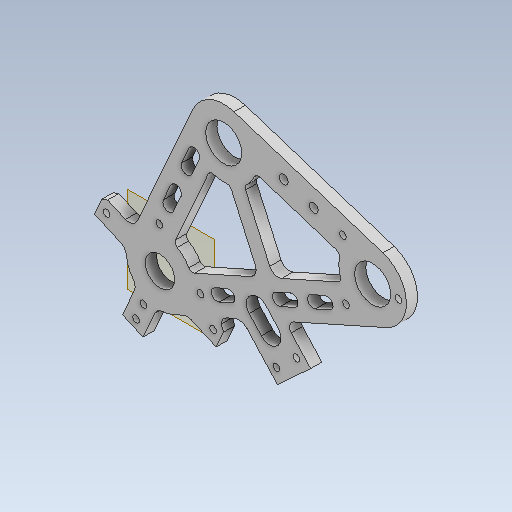
# Autodesk Inventor part: motor_holder_3
Saved by Autodesk Inventor 2020 (Build 240168000, 168)
## iProperties
Created: 2020-05-09
Part Number: motor_holder_3
Material: Generic
Document SubType Name: Modeling
Designer: psrobotics
Density: 1 g/cm^3
Appearance: Default
Author: psrobotics
Autodesk Inventor part; units mm, degrees
ref_plane "YZ Plane" through (0, 0, 0) normal (1, 0, 0) x (0, 1, 0)
ref_plane "XZ Plane" through (0, 0, 0) normal (0, 1, 0) x (-1, 0, 0)
ref_plane "XY Plane" through (0, 0, 0) normal (0, 0, 1) x (1, 0, 0)
ref_plane "Work Plane1" through (0, 0, 3) normal (0, 0, 1) x (1, 0, 0)
sketch "Sketch1" plane through (0, 0, 3) normal (0, 0, 1) x (1, 0, 0)
  circle A0 centre (0, 0) radius 4.075 projected
  circle A1 centre (28.3096, 63.473) radius 5.075 projected
  circle A2 centre (94.4874, 42.242) radius 5.075 projected
  line L0 (0, 0) -> (28.3096, 63.473)
  line L1 (28.3096, 63.473) -> (94.4874, 42.242)
  line L2 (94.4874, 42.242) -> (0, 0)
  line L3 (0, 0) -> (28.3096, 63.473) construction
  line L4 (13.6992, -6.11) -> (42.0088, 57.363)
  line L5 (14.6104, 69.5829) -> (-13.6992, 6.11)
  arc A3 (-13.6992, 6.11) -> (13.6992, -6.11) centre (0, 0) ccw
  arc A4 (42.0088, 57.363) -> (14.6104, 69.5829) centre (28.3096, 63.473) ccw
  line L6 (28.3096, 63.473) -> (94.4874, 42.242) construction
  line L7 (23.7274, 49.19) -> (89.9052, 27.959)
  line L8 (99.0696, 56.525) -> (32.8918, 77.7559)
  arc A5 (32.8918, 77.7559) -> (23.7274, 49.19) centre (28.3096, 63.473) ccw
  arc A6 (89.9052, 27.959) -> (99.0696, 56.525) centre (94.4874, 42.242) ccw
  line L9 (94.4874, 42.242) -> (0, 0) construction
  line L10 (88.3654, 55.9358) -> (-6.122, 13.6938)
  line L11 (6.122, -13.6938) -> (100.6094, 28.5482)
  arc A7 (100.6094, 28.5482) -> (88.3654, 55.9358) centre (94.4874, 42.242) ccw
  arc A8 (-6.122, 13.6938) -> (6.122, -13.6938) centre (0, 0) ccw
  circle A9 centre (0, 0) radius 15
  circle A10 centre (28.3096, 63.473) radius 15
  circle A11 centre (94.4874, 42.242) radius 15
  point P0 (0, 0)
  point P1 (14.1548, 31.7365)
  point P2 (61.3985, 52.8575)
  point P3 (47.2437, 21.121)
  point P4 (13.6938, 6.122)
  point P5 (6.11, 13.6992)
  point P6 (22.1996, 49.7738)
  point P7 (23.7274, 49.19)
  point P8 (42.5926, 58.8907)
  point P9 (80.2044, 46.8242)
  point P10 (80.7936, 36.12)
  point P11 (32.8918, 77.7559)
  point P12 (6.122, -13.6938)
  dimension "d0" = 30
  dimension "d1" = 30
  dimension "d2" = 30
  dimension "d3" = 30
  dimension "d4" = 30
  dimension "d5" = 30
  constraints: 30 end point, 12 point on circle, 12 tangent, 9 centre point, 5 equal length, 3 coincident, 3 midpoint, 1 concentric, 1 point on line
  measures "d0" diameter of A4
  measures "d1" diameter of A6
  measures "d2" diameter of A8
  measures "d3" diameter of A9
  measures "d4" diameter of A10
  measures "d5" diameter of A11
extrude "Extrusion1" add sketch "Sketch1" along normal blind 5 contours A0 L0 L2 | A0 L2 A9 A3 A8 L0 | L2 L0 A0 | A0 L0 A9 L2 | L2 L4 A9 | A9 L10 L0 | L2 L7 A6 L11 A3 L4 | L10 A8 L5 A5 L0 | L2 A11 L7 | A5 A4 L1 A1 L0 | L0 A1 L1 A4 A10 A5 | A11 L1 A2 L2 | L2 A2 L1 A11 A7 A6 | L0 L1 A1 | A1 L1 L0 | L2 L1 A2 | A2 L1 L2 | L1 L10 A11 | L1 A4 L8 A7 L10
sketch "Sketch2" plane through (0, 0, 8) normal (0, 0, 1) x (1, 0, 0)
  line L0 (52.1909, -17.5786) -> (66.9432, -4.074) projected
  line L1 (66.9432, -4.074) -> (60.1909, 3.3021) projected
  line L2 (45.4387, -10.2024) -> (52.1909, -17.5786) projected
  arc A0 (-13.6992, 6.11) -> (6.122, -13.6938) centre (0, 0) ccw projected
  line L3 (6.122, -13.6938) -> (100.6094, 28.5482) projected
  arc A1 (100.6094, 28.5482) -> (99.0696, 56.525) centre (94.4874, 42.242) ccw projected
  line L4 (99.0696, 56.525) -> (32.8918, 77.7559) projected
  arc A2 (32.8918, 77.7559) -> (14.6104, 69.5829) centre (28.3096, 63.473) ccw projected
  line L5 (14.6104, 69.5829) -> (-13.6992, 6.11) projected
  arc A3 (22.1996, 49.7738) -> (42.5926, 58.8907) centre (28.3096, 63.473) ccw projected
  line L6 (42.5926, 58.8907) -> (80.2044, 46.8242) projected
  arc A4 (80.2044, 46.8242) -> (80.7936, 36.12) centre (94.4874, 42.242) ccw projected
  line L7 (80.7936, 36.12) -> (13.6938, 6.122) projected
  arc A5 (13.6938, 6.122) -> (6.11, 13.6992) centre (0, 0) ccw projected
  line L8 (6.11, 13.6992) -> (22.1996, 49.7738) projected
  line L9 (47.4643, -12.4153) -> (36.2889, -0.2073)
  line L10 (6.122, -13.6938) -> (100.6094, 28.5482) projected
  line L11 (62.2166, 1.0892) -> (55.5293, 8.3944)
  circle A6 centre (60.6166, -3.0869) radius 2.05 projected
  circle A7 centre (51.7652, -11.1896) radius 2.05 projected
  line L12 (60.1909, 3.3021) -> (45.4387, -10.2024) projected
  point P0 (0, 0)
  point P1 (36.2889, -0.2073)
  constraints: 4 end point, 2 point on line, 1 parallel
extrude "Extrusion2" add sketch "Sketch2" against normal blind 5 contours L2 L12 L1 L0 | L9 L3 L11 L12 | A6 | A7
sketch "Sketch3" plane through (0, 0, 8) normal (0, 0, 1) x (1, 0, 0)
  circle A0 centre (60.6166, -3.0869) radius 2.05 projected
  circle A1 centre (51.7652, -11.1896) radius 2.05 projected
  point P0 (0, 0)
hole "Hole1" at (60.6166, -3.0869, 8) at (51.7652, -11.1896, 8) direction (0, 0, -1) diameter 3 depth 17
sketch "Sketch4" plane through (0, 0, 8) normal (0, 0, 1) x (1, 0, 0)
  line L0 (-20.0514, 14.2904) -> (-19.0396, 11.6492) projected
  line L1 (-20.0514, 14.2904) -> (-23.2479, 15.7161) projected
  line L2 (-25.8892, 14.7042) -> (-23.2479, 15.7161) projected
  line L3 (-25.8892, 14.7042) -> (-29.1478, 7.3979) projected
  arc A0 (-26.4298, 1.9282) -> (-29.1478, 7.3979) centre (-32.4139, 2.3648) ccw projected
  arc A1 (-26.4298, 1.9282) -> (-18.3105, -19.1566) centre (0, 0) ccw projected
  arc A2 (-16.6845, -25.1334) -> (-18.3105, -19.1566) centre (-22.4562, -23.494) ccw projected
  line L4 (-16.6845, -25.1334) -> (-7.5517, -29.2067) projected
  arc A3 (-2.0186, -26.423) -> (-7.5517, -29.2067) centre (-2.4756, -32.4056) ccw projected
  arc A4 (-2.0186, -26.423) -> (19.0939, -18.3759) centre (0, 0) ccw projected
  arc A5 (24.9796, -16.7435) -> (19.0939, -18.3759) centre (23.4171, -22.5364) ccw projected
  line L5 (24.9796, -16.7435) -> (28.2383, -9.4372) projected
  line L6 (27.2264, -6.796) -> (28.2383, -9.4372) projected
  line L7 (27.2264, -6.796) -> (24.0299, -5.3703) projected
  line L8 (21.3887, -6.3822) -> (24.0299, -5.3703) projected
  line L9 (21.3887, -6.3822) -> (18.5667, -12.7093) projected
  arc A6 (-21.8615, 5.3221) -> (18.5667, -12.7093) centre (0, 0) ccw projected
  line L10 (-21.8615, 5.3221) -> (-19.0396, 11.6492) projected
  circle A7 centre (-23.6864, 10.4368) radius 2.075 projected
  circle A8 centre (23.5915, -10.6496) radius 2.075 projected
  circle A9 centre (-10.5906, -23.7453) radius 2.075 projected
  line L11 (22.2033, -4.5557) -> (29.0529, -7.6107)
  line L12 (29.0529, -7.6107) -> (24.9796, -16.7435)
  line L13 (24.9796, -16.7435) -> (18.13, -13.6885)
  line L14 (18.13, -13.6885) -> (22.2033, -4.5557)
  line L15 (22.2033, -4.5557) -> (24.9796, -16.7435) construction
  line L16 (29.0529, -7.6107) -> (18.13, -13.6885) construction
  circle A10 centre (60.6166, -3.0869) radius 1.5 projected
  circle A11 centre (51.7652, -11.1896) radius 1.5 projected
  line L17 (99.0696, 56.525) -> (32.8918, 77.7559) projected
  arc A12 (32.8918, 77.7559) -> (14.6104, 69.5829) centre (28.3096, 63.473) ccw projected
  line L18 (14.6104, 69.5829) -> (-13.6992, 6.11) projected
  arc A13 (-13.6992, 6.11) -> (6.122, -13.6938) centre (0, 0) ccw projected
  line L19 (6.122, -13.6938) -> (36.2889, -0.2073) projected
  line L20 (36.2889, -0.2073) -> (52.1909, -17.5786) projected
  line L21 (52.1909, -17.5786) -> (66.9432, -4.074) projected
  line L22 (66.9432, -4.074) -> (55.5293, 8.3944) projected
  line L23 (55.5293, 8.3944) -> (100.6094, 28.5482) projected
  arc A14 (100.6094, 28.5482) -> (99.0696, 56.525) centre (94.4874, 42.242) ccw projected
  line L24 (6.11, 13.6992) -> (22.1996, 49.7738) projected
  arc A15 (22.1996, 49.7738) -> (42.5926, 58.8907) centre (28.3096, 63.473) ccw projected
  line L25 (42.5926, 58.8907) -> (80.2044, 46.8242) projected
  arc A16 (80.2044, 46.8242) -> (80.7936, 36.12) centre (94.4874, 42.242) ccw projected
  line L26 (80.7936, 36.12) -> (13.6938, 6.122) projected
  arc A17 (13.6938, 6.122) -> (6.11, 13.6992) centre (0, 0) ccw projected
  line L27 (18.13, -13.6885) -> (12.1249, -11.0101)
  line L28 (6.122, -13.6938) -> (36.2889, -0.2073) projected
  point P0 (0, 0)
  point P1 (28.2382, -9.4374)
  point P2 (24.3854, -5.5289)
  dimension "d17" = 7.5
  dimension "d18" = 10
  constraints: 14 end point, 2 collinear, 2 midpoint, 2 parallel, 1 perpendicular, 1 point on line
  measures "d17" distance of L11.start L11.end
  measures "d18" distance of L11.end L12.end
extrude "Extrusion3" add sketch "Sketch4" against normal blind 5 contours L27 L19 L9 A6 | A6 L14 L27 | L9 L19 L7 L6 L5 L13 L14 | L6 L11 L12
sketch "Sketch5" plane through (0, 0, 8) normal (0, 0, 1) x (1, 0, 0)
  circle A0 centre (-10.5906, -23.7453) radius 2.075 projected
  circle A1 centre (-23.6864, 10.4368) radius 2.075 projected
  line L0 (-20.0514, 14.2904) -> (-19.0396, 11.6492) projected
  line L1 (-20.0514, 14.2904) -> (-23.2479, 15.7161) projected
  line L2 (-25.8892, 14.7042) -> (-23.2479, 15.7161) projected
  line L3 (-25.8892, 14.7042) -> (-29.1478, 7.3979) projected
  arc A2 (-26.4298, 1.9282) -> (-29.1478, 7.3979) centre (-32.4139, 2.3648) ccw projected
  arc A3 (-26.4298, 1.9282) -> (-18.3105, -19.1566) centre (0, 0) ccw projected
  arc A4 (-16.6845, -25.1334) -> (-18.3105, -19.1566) centre (-22.4562, -23.494) ccw projected
  line L4 (-16.6845, -25.1334) -> (-7.5517, -29.2067) projected
  arc A5 (-2.0186, -26.423) -> (-7.5517, -29.2067) centre (-2.4756, -32.4056) ccw projected
  arc A6 (-2.0186, -26.423) -> (19.0939, -18.3759) centre (0, 0) ccw projected
  arc A7 (24.9796, -16.7435) -> (19.0939, -18.3759) centre (23.4171, -22.5364) ccw projected
  line L5 (24.9796, -16.7435) -> (28.2383, -9.4372) projected
  line L6 (27.2264, -6.796) -> (28.2383, -9.4372) projected
  line L7 (27.2264, -6.796) -> (24.0299, -5.3703) projected
  line L8 (21.3887, -6.3822) -> (24.0299, -5.3703) projected
  line L9 (21.3887, -6.3822) -> (18.5667, -12.7093) projected
  arc A8 (-21.8615, 5.3221) -> (18.5667, -12.7093) centre (0, 0) ccw projected
  line L10 (-21.8615, 5.3221) -> (-19.0396, 11.6492) projected
  circle A9 centre (-23.6864, 10.4368) radius 2.075 projected
  circle A10 centre (23.5915, -10.6496) radius 2.075 projected
  circle A11 centre (-10.5906, -23.7453) radius 2.075 projected
  line L11 (-4.4968, -22.3571) -> (-7.5517, -29.2067)
  line L12 (-7.5517, -29.2067) -> (-16.6845, -25.1334)
  line L13 (-16.6845, -25.1334) -> (-13.6296, -18.2838)
  line L14 (-13.6296, -18.2838) -> (-4.4968, -22.3571)
  line L15 (-4.4968, -22.3571) -> (-16.6845, -25.1334) construction
  line L16 (-7.5517, -29.2067) -> (-13.6296, -18.2838) construction
  line L17 (-18.2249, 13.4757) -> (-25.0745, 16.5307)
  line L18 (-25.0745, 16.5307) -> (-29.1478, 7.3979)
  line L19 (-29.1478, 7.3979) -> (-22.2982, 4.3429)
  line L20 (-22.2982, 4.3429) -> (-18.2249, 13.4757)
  line L21 (-18.2249, 13.4757) -> (-29.1478, 7.3979) construction
  line L22 (-25.0745, 16.5307) -> (-22.2982, 4.3429) construction
  circle A12 centre (23.5915, -10.6496) radius 2.075 projected
  circle A13 centre (60.6166, -3.0869) radius 1.5 projected
  circle A14 centre (51.7652, -11.1896) radius 1.5 projected
  line L23 (99.0696, 56.525) -> (32.8918, 77.7559) projected
  arc A15 (32.8918, 77.7559) -> (14.6104, 69.5829) centre (28.3096, 63.473) ccw projected
  line L24 (14.6104, 69.5829) -> (-13.6992, 6.11) projected
  arc A16 (-13.6992, 6.11) -> (6.122, -13.6938) centre (0, 0) ccw projected
  line L25 (6.122, -13.6938) -> (12.1249, -11.0101) projected
  line L26 (12.1249, -11.0101) -> (24.9796, -16.7435) projected
  line L27 (24.9796, -16.7435) -> (29.0529, -7.6107) projected
  line L28 (29.0529, -7.6107) -> (24.3854, -5.5289) projected
  line L29 (24.3854, -5.5289) -> (36.2889, -0.2073) projected
  line L30 (36.2889, -0.2073) -> (52.1909, -17.5786) projected
  line L31 (52.1909, -17.5786) -> (66.9432, -4.074) projected
  line L32 (66.9432, -4.074) -> (55.5293, 8.3944) projected
  line L33 (55.5293, 8.3944) -> (100.6094, 28.5482) projected
  arc A17 (100.6094, 28.5482) -> (99.0696, 56.525) centre (94.4874, 42.242) ccw projected
  line L34 (6.11, 13.6992) -> (22.1996, 49.7738) projected
  arc A18 (22.1996, 49.7738) -> (42.5926, 58.8907) centre (28.3096, 63.473) ccw projected
  line L35 (42.5926, 58.8907) -> (80.2044, 46.8242) projected
  arc A19 (80.2044, 46.8242) -> (80.7936, 36.12) centre (94.4874, 42.242) ccw projected
  line L36 (80.7936, 36.12) -> (13.6938, 6.122) projected
  arc A20 (13.6938, 6.122) -> (6.11, 13.6992) centre (0, 0) ccw projected
  line L37 (-4.4968, -22.3571) -> (-1.1942, -14.9524)
  arc A21 (-13.6992, 6.11) -> (6.122, -13.6938) centre (0, 0) ccw projected
  line L38 (-13.6296, -18.2838) -> (-10.327, -10.8791)
  line L39 (-22.2982, 4.3429) -> (-14.9617, 1.0708)
  line L40 (-18.2249, 13.4757) -> (-11.71, 10.57)
  point P0 (0, 0)
  dimension "d21" = 7.5
  dimension "d22" = 10
  dimension "d23" = 7.5
  dimension "d24" = 10
  constraints: 32 end point, 6 collinear, 4 midpoint, 4 parallel, 3 point on circle, 2 perpendicular, 1 point on line
  measures "d21" distance of L11.start L11.end
  measures "d22" distance of L11.end L12.end
  measures "d23" distance of L17.start L17.end
  measures "d24" distance of L18.end L17.end
extrude "Extrusion4" add sketch "Sketch5" against normal blind 5 contours L17 L20 L0 | L0 L10 L20 L19 L3 L2 L1 | L20 L40 L24 A16 L39 A8 L10 | L2 L18 L17 | A8 L39 L20 | L38 A16 L37 A8 L14 | A8 L14 L38 | L14 A8 | A8 L14 L11 L4 L13 | A8 L37 L14
chamfer "Chamfer1" distance 2 angle 45 2 edges at (-25.0745, 16.5307, 5.5) (29.0529, -7.6107, 5.5)
sketch "Sketch6" plane through (0, 0, 8) normal (0, 0, 1) x (1, 0, 0)
  line L0 (27.2264, -6.796) -> (28.2383, -9.4372) projected
  line L1 (27.2264, -6.796) -> (24.3854, -5.5289) projected
  line L2 (24.3854, -5.5289) -> (36.2889, -0.2073) projected
  line L3 (36.2889, -0.2073) -> (52.1909, -17.5786) projected
  line L4 (52.1909, -17.5786) -> (66.9432, -4.074) projected
  line L5 (66.9432, -4.074) -> (55.5293, 8.3944) projected
  line L6 (55.5293, 8.3944) -> (100.6094, 28.5482) projected
  arc A0 (100.6094, 28.5482) -> (99.0696, 56.525) centre (94.4874, 42.242) ccw projected
  line L7 (99.0696, 56.525) -> (32.8918, 77.7559) projected
  arc A1 (32.8918, 77.7559) -> (14.6104, 69.5829) centre (28.3096, 63.473) ccw projected
  line L8 (14.6104, 69.5829) -> (-11.71, 10.57) projected
  line L9 (-11.71, 10.57) -> (-23.2479, 15.7161) projected
  line L10 (-25.8892, 14.7042) -> (-23.2479, 15.7161) projected
  line L11 (-25.8892, 14.7042) -> (-29.1478, 7.3979) projected
  line L12 (-29.1478, 7.3979) -> (-14.9617, 1.0708) projected
  arc A2 (-14.9617, 1.0708) -> (-10.327, -10.8791) centre (0, 0) ccw projected
  line L13 (-10.327, -10.8791) -> (-16.6845, -25.1334) projected
  line L14 (-16.6845, -25.1334) -> (-7.5517, -29.2067) projected
  line L15 (-7.5517, -29.2067) -> (-1.1942, -14.9524) projected
  arc A3 (-1.1942, -14.9524) -> (6.122, -13.6938) centre (0, 0) ccw projected
  line L16 (6.122, -13.6938) -> (12.1249, -11.0101) projected
  line L17 (12.1249, -11.0101) -> (24.9796, -16.7435) projected
  line L18 (24.9796, -16.7435) -> (28.2383, -9.4372) projected
  circle A4 centre (-23.6864, 10.4368) radius 2.075 projected
  circle A5 centre (-10.5906, -23.7453) radius 2.075 projected
  circle A6 centre (23.5915, -10.6496) radius 2.075 projected
  circle A7 centre (60.6166, -3.0869) radius 1.5 projected
  circle A8 centre (51.7652, -11.1896) radius 1.5 projected
  line L19 (6.11, 13.6992) -> (22.1996, 49.7738) projected
  arc A9 (22.1996, 49.7738) -> (42.5926, 58.8907) centre (28.3096, 63.473) ccw projected
  line L20 (42.5926, 58.8907) -> (80.2044, 46.8242) projected
  arc A10 (80.2044, 46.8242) -> (80.7936, 36.12) centre (94.4874, 42.242) ccw projected
  line L21 (80.7936, 36.12) -> (13.6938, 6.122) projected
  arc A11 (13.6938, 6.122) -> (6.11, 13.6992) centre (0, 0) ccw projected
  circle A12 centre (23.5915, -10.6496) radius 2.075 projected
  circle A13 centre (23.5915, -10.6496) radius 1.5
  circle A14 centre (-10.5906, -23.7453) radius 2.075 projected
  circle A15 centre (-10.5906, -23.7453) radius 1.5
  circle A16 centre (-23.6864, 10.4368) radius 1.5
  point P0 (0, 0)
  dimension "d30" = 3
  dimension "d31" = 3
  dimension "d32" = 3
  constraints: 3 centre point, 3 coincident
  measures "d30" diameter of A13
  measures "d31" diameter of A15
  measures "d32" diameter of A16
extrude "Extrusion5" add sketch "Sketch6" against normal up to surface (5 mm away) contours A4 | A5 | A6
fillet "Fillet1" radius 4 6 edges at (24.3854, -5.5289, 5.5) (12.1249, -11.0101, 5.5) (-1.1942, -14.9524, 5.5) (-10.327, -10.8791, 5.5) (-14.9617, 1.0708, 5.5) (-11.71, 10.57, 5.5)
sketch "Sketch7" plane through (0, 0, 8) normal (0, 0, 1) x (1, 0, 0)
  circle A0 centre (-23.6864, 10.4368) radius 1.5 projected
  circle A1 centre (23.5915, -10.6496) radius 1.5 projected
  circle A2 centre (-10.5906, -23.7453) radius 1.5 projected
  line L0 (27.2264, -6.796) -> (28.2383, -9.4372) projected
  arc A3 (29.5934, -3.2006) -> (27.2264, -6.796) centre (31.226, -6.8523) ccw projected
  line L1 (29.5934, -3.2006) -> (36.2889, -0.2073) projected
  line L2 (36.2889, -0.2073) -> (52.1909, -17.5786) projected
  line L3 (52.1909, -17.5786) -> (66.9432, -4.074) projected
  line L4 (66.9432, -4.074) -> (55.5293, 8.3944) projected
  line L5 (55.5293, 8.3944) -> (100.6094, 28.5482) projected
  arc A4 (100.6094, 28.5482) -> (99.0696, 56.525) centre (94.4874, 42.242) ccw projected
  line L6 (99.0696, 56.525) -> (32.8918, 77.7559) projected
  arc A5 (32.8918, 77.7559) -> (14.6104, 69.5829) centre (28.3096, 63.473) ccw projected
  line L7 (14.6104, 69.5829) -> (-10.0806, 14.2231) projected
  arc A6 (-15.3631, 12.1994) -> (-10.0806, 14.2231) centre (-13.7338, 15.8525) ccw projected
  line L8 (-15.3631, 12.1994) -> (-23.2479, 15.7161) projected
  line L9 (-25.8892, 14.7042) -> (-23.2479, 15.7161) projected
  line L10 (-25.8892, 14.7042) -> (-29.1478, 7.3979) projected
  line L11 (-29.1478, 7.3979) -> (-17.3085, 2.1175) projected
  arc A7 (-14.9509, -1.2123) -> (-17.3085, 2.1175) centre (-18.9378, -1.5356) ccw projected
  arc A8 (-14.9509, -1.2123) -> (-11.8701, -9.1706) centre (0, 0) ccw projected
  arc A9 (-11.3824, -13.2454) -> (-11.8701, -9.1706) centre (-15.0355, -11.6161) ccw projected
  line L12 (-11.3824, -13.2454) -> (-16.6845, -25.1334) projected
  line L13 (-16.6845, -25.1334) -> (-7.5517, -29.2067) projected
  line L14 (-7.5517, -29.2067) -> (-2.2496, -17.3188) projected
  arc A10 (1.1081, -14.959) -> (-2.2496, -17.3188) centre (1.4035, -18.9481) ccw projected
  arc A11 (1.1081, -14.959) -> (6.122, -13.6938) centre (0, 0) ccw projected
  line L15 (6.122, -13.6938) -> (10.4943, -11.7391) projected
  arc A12 (13.7562, -11.7377) -> (10.4943, -11.7391) centre (12.1268, -15.3908) ccw projected
  line L16 (13.7562, -11.7377) -> (24.9796, -16.7435) projected
  line L17 (24.9796, -16.7435) -> (28.2383, -9.4372) projected
  circle A13 centre (60.6166, -3.0869) radius 1.5 projected
  circle A14 centre (51.7652, -11.1896) radius 1.5 projected
  line L18 (6.11, 13.6992) -> (22.1996, 49.7738) projected
  arc A15 (22.1996, 49.7738) -> (42.5926, 58.8907) centre (28.3096, 63.473) ccw projected
  line L19 (42.5926, 58.8907) -> (80.2044, 46.8242) projected
  arc A16 (80.2044, 46.8242) -> (80.7936, 36.12) centre (94.4874, 42.242) ccw projected
  line L20 (80.7936, 36.12) -> (13.6938, 6.122) projected
  arc A17 (13.6938, 6.122) -> (6.11, 13.6992) centre (0, 0) ccw projected
  line L21 (28.3096, 63.473) -> (47.2437, 21.121)
  line L22 (80.7936, 36.12) -> (13.6938, 6.122) projected
  line L23 (44.7848, 18.0455) -> (51.1753, 20.9024)
  line L24 (51.1753, 20.9024) -> (30.7685, 66.5485)
  line L25 (30.7685, 66.5485) -> (24.3781, 63.6915)
  line L26 (24.3781, 63.6915) -> (44.7848, 18.0455)
  line L27 (44.7848, 18.0455) -> (30.7685, 66.5485) construction
  line L28 (51.1753, 20.9024) -> (24.3781, 63.6915) construction
  point P0 (0, 0)
  point P1 (37.7767, 42.297)
  point P2 (31.0674, 48.7286)
  point P3 (44.0485, 19.6925)
  point P4 (50.4389, 22.5495)
  point P5 (37.4579, 51.5856)
  dimension "d36" = 7
  dimension "d37" = 50
  constraints: 14 end point, 4 midpoint, 2 parallel, 2 perpendicular
  measures "d36" distance of L23.start L23.end
  measures "d37" distance of L24.end L23.end
extrude "Extrusion6" add sketch "Sketch7" against normal blind 5 contours A15 L21 L20 L26 | A15 L24 L20 L21
sketch "Sketch8" plane through (0, 0, 8) normal (0, 0, 1) x (1, 0, 0)
  circle A0 centre (68.3193, 58.5137) radius 1.5 projected
  circle A1 centre (54.9885, 62.7904) radius 1.5 projected
  circle A2 centre (54.9885, 62.7904) radius 2
  circle A3 centre (68.3193, 58.5137) radius 2
  point P0 (0, 0)
  dimension "d40" = 4
  dimension "d41" = 4
  constraints: 2 centre point, 2 coincident
  measures "d40" diameter of A2
  measures "d41" diameter of A3
extrude "Extrusion7" cut sketch "Sketch8" against normal blind 5 contours A0 | A1 | A2 | A3
sketch "Sketch9" plane through (0, 0, 8) normal (0, 0, 1) x (1, 0, 0)
  circle A0 centre (54.9885, 62.7904) radius 2 projected
  circle A1 centre (68.3193, 58.5137) radius 2 projected
  arc A2 (37.4579, 51.5856) -> (42.5926, 58.8907) centre (28.3096, 63.473) ccw projected
  line L0 (42.5926, 58.8907) -> (80.2044, 46.8242) projected
  arc A3 (80.2044, 46.8242) -> (80.7936, 36.12) centre (94.4874, 42.242) ccw projected
  line L1 (80.7936, 36.12) -> (50.4389, 22.5495) projected
  line L2 (50.4389, 22.5495) -> (37.4579, 51.5856) projected
  circle A4 centre (-23.6864, 10.4368) radius 1.5 projected
  circle A5 centre (23.5915, -10.6496) radius 1.5 projected
  circle A6 centre (-10.5906, -23.7453) radius 1.5 projected
  circle A7 centre (60.6166, -3.0869) radius 1.5 projected
  circle A8 centre (51.7652, -11.1896) radius 1.5 projected
  line L3 (27.2264, -6.796) -> (28.2383, -9.4372) projected
  arc A9 (29.5934, -3.2006) -> (27.2264, -6.796) centre (31.226, -6.8523) ccw projected
  line L4 (29.5934, -3.2006) -> (36.2889, -0.2073) projected
  line L5 (36.2889, -0.2073) -> (52.1909, -17.5786) projected
  line L6 (52.1909, -17.5786) -> (66.9432, -4.074) projected
  line L7 (66.9432, -4.074) -> (55.5293, 8.3944) projected
  line L8 (55.5293, 8.3944) -> (100.6094, 28.5482) projected
  arc A10 (100.6094, 28.5482) -> (99.0696, 56.525) centre (94.4874, 42.242) ccw projected
  line L9 (99.0696, 56.525) -> (32.8918, 77.7559) projected
  arc A11 (32.8918, 77.7559) -> (14.6104, 69.5829) centre (28.3096, 63.473) ccw projected
  line L10 (14.6104, 69.5829) -> (-10.0806, 14.2231) projected
  arc A12 (-15.3631, 12.1994) -> (-10.0806, 14.2231) centre (-13.7338, 15.8525) ccw projected
  line L11 (-15.3631, 12.1994) -> (-23.2479, 15.7161) projected
  line L12 (-25.8892, 14.7042) -> (-23.2479, 15.7161) projected
  line L13 (-25.8892, 14.7042) -> (-29.1478, 7.3979) projected
  line L14 (-29.1478, 7.3979) -> (-17.3085, 2.1175) projected
  arc A13 (-14.9509, -1.2123) -> (-17.3085, 2.1175) centre (-18.9378, -1.5356) ccw projected
  arc A14 (-14.9509, -1.2123) -> (-11.8701, -9.1706) centre (0, 0) ccw projected
  arc A15 (-11.3824, -13.2454) -> (-11.8701, -9.1706) centre (-15.0355, -11.6161) ccw projected
  line L15 (-11.3824, -13.2454) -> (-16.6845, -25.1334) projected
  line L16 (-16.6845, -25.1334) -> (-7.5517, -29.2067) projected
  line L17 (-7.5517, -29.2067) -> (-2.2496, -17.3188) projected
  arc A16 (1.1081, -14.959) -> (-2.2496, -17.3188) centre (1.4035, -18.9481) ccw projected
  arc A17 (1.1081, -14.959) -> (6.122, -13.6938) centre (0, 0) ccw projected
  line L18 (6.122, -13.6938) -> (10.4943, -11.7391) projected
  arc A18 (13.7562, -11.7377) -> (10.4943, -11.7391) centre (12.1268, -15.3908) ccw projected
  line L19 (13.7562, -11.7377) -> (24.9796, -16.7435) projected
  line L20 (24.9796, -16.7435) -> (28.2383, -9.4372) projected
  line L21 (31.0674, 48.7286) -> (44.0485, 19.6925) projected
  line L22 (44.0485, 19.6925) -> (13.6938, 6.122) projected
  arc A19 (13.6938, 6.122) -> (6.11, 13.6992) centre (0, 0) ccw projected
  line L23 (6.11, 13.6992) -> (22.1996, 49.7738) projected
  arc A20 (22.1996, 49.7738) -> (31.0674, 48.7286) centre (28.3096, 63.473) ccw projected
  circle A21 centre (94.4874, 42.242) radius 8
  circle A22 centre (28.3096, 63.473) radius 8
  point P0 (0, 0)
  dimension "d44" = 16
  dimension "d45" = 16
  constraints: 2 centre point, 2 coincident
  measures "d44" diameter of A21
  measures "d45" diameter of A22
extrude "Extrusion8" cut sketch "Sketch9" against normal blind 10 contours A21 | A22
sketch "Sketch10" plane through (0, 0, 8) normal (0, 0, 1) x (1, 0, 0)
  circle A0 centre (0, 0) radius 6.5
  dimension "d48" = 13
  constraints: 1 centre point, 1 coincident
  measures "d48" diameter of A0
extrude "Extrusion9" cut sketch "Sketch10" against normal blind 10
sketch "Sketch11" plane through (0, 0, 8) normal (0, 0, 1) x (1, 0, 0)
  circle A0 centre (0, 0) radius 6.5 projected
  circle A1 centre (28.3096, 63.473) radius 8 projected
  circle A2 centre (94.4874, 42.242) radius 8 projected
  circle A3 centre (54.9885, 62.7904) radius 2 projected
  circle A4 centre (68.3193, 58.5137) radius 2 projected
  arc A5 (37.4579, 51.5856) -> (42.5926, 58.8907) centre (28.3096, 63.473) ccw projected
  line L0 (42.5926, 58.8907) -> (80.2044, 46.8242) projected
  arc A6 (80.2044, 46.8242) -> (80.7936, 36.12) centre (94.4874, 42.242) ccw projected
  line L1 (80.7936, 36.12) -> (50.4389, 22.5495) projected
  line L2 (50.4389, 22.5495) -> (37.4579, 51.5856) projected
  circle A7 centre (-23.6864, 10.4368) radius 1.5 projected
  circle A8 centre (23.5915, -10.6496) radius 1.5 projected
  circle A9 centre (-10.5906, -23.7453) radius 1.5 projected
  circle A10 centre (60.6166, -3.0869) radius 1.5 projected
  circle A11 centre (51.7652, -11.1896) radius 1.5 projected
  line L3 (27.2264, -6.796) -> (28.2383, -9.4372) projected
  arc A12 (29.5934, -3.2006) -> (27.2264, -6.796) centre (31.226, -6.8523) ccw projected
  line L4 (29.5934, -3.2006) -> (36.2889, -0.2073) projected
  line L5 (36.2889, -0.2073) -> (52.1909, -17.5786) projected
  line L6 (52.1909, -17.5786) -> (66.9432, -4.074) projected
  line L7 (66.9432, -4.074) -> (55.5293, 8.3944) projected
  line L8 (55.5293, 8.3944) -> (100.6094, 28.5482) projected
  arc A13 (100.6094, 28.5482) -> (99.0696, 56.525) centre (94.4874, 42.242) ccw projected
  line L9 (99.0696, 56.525) -> (32.8918, 77.7559) projected
  arc A14 (32.8918, 77.7559) -> (14.6104, 69.5829) centre (28.3096, 63.473) ccw projected
  line L10 (14.6104, 69.5829) -> (-10.0806, 14.2231) projected
  arc A15 (-15.3631, 12.1994) -> (-10.0806, 14.2231) centre (-13.7338, 15.8525) ccw projected
  line L11 (-15.3631, 12.1994) -> (-23.2479, 15.7161) projected
  line L12 (-25.8892, 14.7042) -> (-23.2479, 15.7161) projected
  line L13 (-25.8892, 14.7042) -> (-29.1478, 7.3979) projected
  line L14 (-29.1478, 7.3979) -> (-17.3085, 2.1175) projected
  arc A16 (-14.9509, -1.2123) -> (-17.3085, 2.1175) centre (-18.9378, -1.5356) ccw projected
  arc A17 (-14.9509, -1.2123) -> (-11.8701, -9.1706) centre (0, 0) ccw projected
  arc A18 (-11.3824, -13.2454) -> (-11.8701, -9.1706) centre (-15.0355, -11.6161) ccw projected
  line L15 (-11.3824, -13.2454) -> (-16.6845, -25.1334) projected
  line L16 (-16.6845, -25.1334) -> (-7.5517, -29.2067) projected
  line L17 (-7.5517, -29.2067) -> (-2.2496, -17.3188) projected
  arc A19 (1.1081, -14.959) -> (-2.2496, -17.3188) centre (1.4035, -18.9481) ccw projected
  arc A20 (1.1081, -14.959) -> (6.122, -13.6938) centre (0, 0) ccw projected
  line L18 (6.122, -13.6938) -> (10.4943, -11.7391) projected
  arc A21 (13.7562, -11.7377) -> (10.4943, -11.7391) centre (12.1268, -15.3908) ccw projected
  line L19 (13.7562, -11.7377) -> (24.9796, -16.7435) projected
  line L20 (24.9796, -16.7435) -> (28.2383, -9.4372) projected
  line L21 (31.0674, 48.7286) -> (44.0485, 19.6925) projected
  line L22 (44.0485, 19.6925) -> (13.6938, 6.122) projected
  arc A22 (13.6938, 6.122) -> (6.11, 13.6992) centre (0, 0) ccw projected
  line L23 (6.11, 13.6992) -> (22.1996, 49.7738) projected
  arc A23 (22.1996, 49.7738) -> (31.0674, 48.7286) centre (28.3096, 63.473) ccw projected
  line L24 (94.4874, 42.242) -> (81.2775, 54.469)
  line L25 (94.4874, 42.242) -> (82.6991, 28.6391)
  circle A24 centre (82.6991, 28.6391) radius 1.5
  circle A25 centre (81.2775, 54.469) radius 1.5
  line L26 (94.4874, 42.242) -> (105.9874, 42.242)
  circle A26 centre (105.9874, 42.242) radius 1.5
  dimension "d51" = 18
  dimension "d52" = 18
  dimension "d53" = 3
  dimension "d54" = 3
  dimension "d55" = 11.5
  dimension "d56" = 3
  dimension "d57" = 25
  dimension "d58" = 25
  constraints: 6 end point, 4 coincident, 3 centre point, 1 horizontal
  measures "d51" distance of L24.start L24.end
  measures "d52" distance of L24.start L25.end
  measures "d53" diameter of A24
  measures "d54" diameter of A25
  measures "d55" distance of L24.start L26.end
  measures "d56" diameter of A26
  measures "d57" angle of L8 L25
  measures "d58" angle of L9 L24
extrude "Extrusion10" cut sketch "Sketch11" against normal blind 10 contours A24 | A25 | A26
sketch "Sketch12" plane through (0, 0, 8) normal (0, 0, 1) x (1, 0, 0)
  circle A0 centre (105.9874, 42.242) radius 1.5 projected
  circle A1 centre (81.2775, 54.469) radius 1.5 projected
  circle A2 centre (82.6991, 28.6391) radius 1.5 projected
  circle A3 centre (0, 0) radius 6.5 projected
  circle A4 centre (28.3096, 63.473) radius 8 projected
  circle A5 centre (94.4874, 42.242) radius 8 projected
  circle A6 centre (54.9885, 62.7904) radius 2 projected
  circle A7 centre (68.3193, 58.5137) radius 2 projected
  arc A8 (37.4579, 51.5856) -> (42.5926, 58.8907) centre (28.3096, 63.473) ccw projected
  line L0 (42.5926, 58.8907) -> (80.2044, 46.8242) projected
  arc A9 (80.2044, 46.8242) -> (80.7936, 36.12) centre (94.4874, 42.242) ccw projected
  line L1 (80.7936, 36.12) -> (50.4389, 22.5495) projected
  line L2 (50.4389, 22.5495) -> (37.4579, 51.5856) projected
  circle A10 centre (-23.6864, 10.4368) radius 1.5 projected
  circle A11 centre (23.5915, -10.6496) radius 1.5 projected
  circle A12 centre (-10.5906, -23.7453) radius 1.5 projected
  circle A13 centre (60.6166, -3.0869) radius 1.5 projected
  circle A14 centre (51.7652, -11.1896) radius 1.5 projected
  line L3 (27.2264, -6.796) -> (28.2383, -9.4372) projected
  arc A15 (29.5934, -3.2006) -> (27.2264, -6.796) centre (31.226, -6.8523) ccw projected
  line L4 (29.5934, -3.2006) -> (36.2889, -0.2073) projected
  line L5 (36.2889, -0.2073) -> (52.1909, -17.5786) projected
  line L6 (52.1909, -17.5786) -> (66.9432, -4.074) projected
  line L7 (66.9432, -4.074) -> (55.5293, 8.3944) projected
  line L8 (55.5293, 8.3944) -> (100.6094, 28.5482) projected
  arc A16 (100.6094, 28.5482) -> (99.0696, 56.525) centre (94.4874, 42.242) ccw projected
  line L9 (99.0696, 56.525) -> (32.8918, 77.7559) projected
  arc A17 (32.8918, 77.7559) -> (14.6104, 69.5829) centre (28.3096, 63.473) ccw projected
  line L10 (14.6104, 69.5829) -> (-10.0806, 14.2231) projected
  arc A18 (-15.3631, 12.1994) -> (-10.0806, 14.2231) centre (-13.7338, 15.8525) ccw projected
  line L11 (-15.3631, 12.1994) -> (-23.2479, 15.7161) projected
  line L12 (-25.8892, 14.7042) -> (-23.2479, 15.7161) projected
  line L13 (-25.8892, 14.7042) -> (-29.1478, 7.3979) projected
  line L14 (-29.1478, 7.3979) -> (-17.3085, 2.1175) projected
  arc A19 (-14.9509, -1.2123) -> (-17.3085, 2.1175) centre (-18.9378, -1.5356) ccw projected
  arc A20 (-14.9509, -1.2123) -> (-11.8701, -9.1706) centre (0, 0) ccw projected
  arc A21 (-11.3824, -13.2454) -> (-11.8701, -9.1706) centre (-15.0355, -11.6161) ccw projected
  line L15 (-11.3824, -13.2454) -> (-16.6845, -25.1334) projected
  line L16 (-16.6845, -25.1334) -> (-7.5517, -29.2067) projected
  line L17 (-7.5517, -29.2067) -> (-2.2496, -17.3188) projected
  arc A22 (1.1081, -14.959) -> (-2.2496, -17.3188) centre (1.4035, -18.9481) ccw projected
  arc A23 (1.1081, -14.959) -> (6.122, -13.6938) centre (0, 0) ccw projected
  line L18 (6.122, -13.6938) -> (10.4943, -11.7391) projected
  arc A24 (13.7562, -11.7377) -> (10.4943, -11.7391) centre (12.1268, -15.3908) ccw projected
  line L19 (13.7562, -11.7377) -> (24.9796, -16.7435) projected
  line L20 (24.9796, -16.7435) -> (28.2383, -9.4372) projected
  line L21 (31.0674, 48.7286) -> (44.0485, 19.6925) projected
  line L22 (44.0485, 19.6925) -> (13.6938, 6.122) projected
  arc A25 (13.6938, 6.122) -> (6.11, 13.6992) centre (0, 0) ccw projected
  line L23 (6.11, 13.6992) -> (22.1996, 49.7738) projected
  arc A26 (22.1996, 49.7738) -> (31.0674, 48.7286) centre (28.3096, 63.473) ccw projected
  line L24 (0, 0) -> (-7.332, -16.439)
  line L25 (0, 0) -> (-0.3024, 17.9975)
  line L26 (0, 0) -> (17.9975, 0.3024)
  line L27 (-11.3824, -13.2454) -> (-16.6845, -25.1334) projected
  dimension "d61" = 18
  dimension "d62" = 18
  dimension "d63" = 18
  dimension "d64" = 155
  dimension "d65" = 115
  constraints: 6 end point, 1 parallel
  measures "d61" distance of L24.start L24.end
  measures "d62" distance of L24.start L25.end
  measures "d63" distance of L24.start L26.end
  measures "d64" angle of L24 L25
  measures "d65" angle of L24 L26
hole "Hole2" at (17.9975, 0.3024, 8) at (-7.332, -16.439, 8) at (-0.3024, 17.9975, 8) direction (0, 0, -1) diameter 3 depth 17
fillet "Fillet2" radius 2 8 edges at (80.7936, 36.12, 5.5) (80.2044, 46.8242, 5.5) (42.5926, 58.8907, 5.5) (37.4579, 51.5856, 5.5) (31.0674, 48.7286, 5.5) (22.1996, 49.7738, 5.5) (6.11, 13.6992, 5.5) (13.6938, 6.122, 5.5)
fillet "Fillet3" radius 4 2 edges at (50.4389, 22.5495, 5.5) (44.0485, 19.6925, 5.5)
fillet "Fillet4" radius 3 1 edges at (55.5293, 8.3944, 5.5)
fillet "Fillet5" radius 5 1 edges at (36.2889, -0.2073, 5.5)
sketch "Sketch13" plane through (0, 0, 8) normal (0, 0, 1) x (1, 0, 0)
  circle A0 centre (-7.332, -16.439) radius 1.5 projected
  circle A1 centre (17.9975, 0.3024) radius 1.5 projected
  circle A2 centre (-0.3024, 17.9975) radius 1.5 projected
  circle A3 centre (105.9874, 42.242) radius 1.5 projected
  circle A4 centre (81.2775, 54.469) radius 1.5 projected
  circle A5 centre (82.6991, 28.6391) radius 1.5 projected
  circle A6 centre (0, 0) radius 6.5 projected
  circle A7 centre (28.3096, 63.473) radius 8 projected
  circle A8 centre (94.4874, 42.242) radius 8 projected
  circle A9 centre (54.9885, 62.7904) radius 2 projected
  circle A10 centre (68.3193, 58.5137) radius 2 projected
  arc A11 (38.5327, 52.4963) -> (41.9543, 57.2422) centre (28.3096, 63.473) ccw projected
  arc A12 (44.3846, 58.3158) -> (41.9543, 57.2422) centre (43.7736, 56.4114) ccw projected
  line L0 (44.3846, 58.3158) -> (78.4124, 47.3991) projected
  arc A13 (79.7645, 45.112) -> (78.4124, 47.3991) centre (77.8015, 45.4947) ccw projected
  arc A14 (79.7645, 45.112) -> (80.1684, 37.7735) centre (94.4874, 42.242) ccw projected
  arc A15 (79.0755, 35.3519) -> (80.1684, 37.7735) centre (78.2592, 37.1777) ccw projected
  line L1 (79.0755, 35.3519) -> (54.0906, 24.182) projected
  arc A16 (48.8064, 26.2012) -> (54.0906, 24.182) centre (52.4581, 27.8337) ccw projected
  line L2 (48.8064, 26.2012) -> (38.07, 50.2164) projected
  arc A17 (38.5327, 52.4963) -> (38.07, 50.2164) centre (39.8958, 51.0327) ccw projected
  circle A18 centre (-23.6864, 10.4368) radius 1.5 projected
  circle A19 centre (23.5915, -10.6496) radius 1.5 projected
  circle A20 centre (-10.5906, -23.7453) radius 1.5 projected
  circle A21 centre (60.6166, -3.0869) radius 1.5 projected
  circle A22 centre (51.7652, -11.1896) radius 1.5 projected
  line L3 (27.2264, -6.796) -> (28.2383, -9.4372) projected
  arc A23 (29.5934, -3.2006) -> (27.2264, -6.796) centre (31.226, -6.8523) ccw projected
  line L4 (29.5934, -3.2006) -> (32.9958, -1.6795) projected
  arc A24 (38.7245, -2.868) -> (32.9958, -1.6795) centre (35.0365, -6.2441) ccw projected
  line L5 (38.7245, -2.868) -> (52.1909, -17.5786) projected
  line L6 (52.1909, -17.5786) -> (66.9432, -4.074) projected
  line L7 (66.9432, -4.074) -> (58.3371, 5.3271) projected
  arc A25 (59.3255, 10.0916) -> (58.3371, 5.3271) centre (60.5499, 7.3528) ccw projected
  line L8 (59.3255, 10.0916) -> (100.6094, 28.5482) projected
  arc A26 (100.6094, 28.5482) -> (99.0696, 56.525) centre (94.4874, 42.242) ccw projected
  line L9 (99.0696, 56.525) -> (32.8918, 77.7559) projected
  arc A27 (32.8918, 77.7559) -> (14.6104, 69.5829) centre (28.3096, 63.473) ccw projected
  line L10 (14.6104, 69.5829) -> (-10.0806, 14.2231) projected
  arc A28 (-15.3631, 12.1994) -> (-10.0806, 14.2231) centre (-13.7338, 15.8525) ccw projected
  line L11 (-15.3631, 12.1994) -> (-23.2479, 15.7161) projected
  line L12 (-25.8892, 14.7042) -> (-23.2479, 15.7161) projected
  line L13 (-25.8892, 14.7042) -> (-29.1478, 7.3979) projected
  line L14 (-29.1478, 7.3979) -> (-17.3085, 2.1175) projected
  arc A29 (-14.9509, -1.2123) -> (-17.3085, 2.1175) centre (-18.9378, -1.5356) ccw projected
  arc A30 (-14.9509, -1.2123) -> (-11.8701, -9.1706) centre (0, 0) ccw projected
  arc A31 (-11.3824, -13.2454) -> (-11.8701, -9.1706) centre (-15.0355, -11.6161) ccw projected
  line L15 (-11.3824, -13.2454) -> (-16.6845, -25.1334) projected
  line L16 (-16.6845, -25.1334) -> (-7.5517, -29.2067) projected
  line L17 (-7.5517, -29.2067) -> (-2.2496, -17.3188) projected
  arc A32 (1.1081, -14.959) -> (-2.2496, -17.3188) centre (1.4035, -18.9481) ccw projected
  arc A33 (1.1081, -14.959) -> (6.122, -13.6938) centre (0, 0) ccw projected
  line L18 (6.122, -13.6938) -> (10.4943, -11.7391) projected
  arc A34 (13.7562, -11.7377) -> (10.4943, -11.7391) centre (12.1268, -15.3908) ccw projected
  line L19 (13.7562, -11.7377) -> (24.9796, -16.7435) projected
  line L20 (24.9796, -16.7435) -> (28.2383, -9.4372) projected
  line L21 (31.6795, 47.3595) -> (42.4159, 23.3442) projected
  arc A35 (40.3968, 18.06) -> (42.4159, 23.3442) centre (38.7642, 21.7117) ccw projected
  line L22 (40.3968, 18.06) -> (15.4119, 6.8901) projected
  arc A36 (12.8785, 7.6905) -> (15.4119, 6.8901) centre (14.5956, 8.716) ccw projected
  arc A37 (12.8785, 7.6905) -> (7.6792, 12.8852) centre (0, 0) ccw projected
  arc A38 (6.8766, 15.4179) -> (7.6792, 12.8852) centre (8.7031, 14.6033) ccw projected
  line L23 (6.8766, 15.4179) -> (21.4331, 48.055) projected
  arc A39 (23.8537, 49.1501) -> (21.4331, 48.055) centre (23.2596, 47.2403) ccw projected
  arc A40 (23.8537, 49.1501) -> (29.672, 48.535) centre (28.3096, 63.473) ccw projected
  arc A41 (31.6795, 47.3595) -> (29.672, 48.535) centre (29.8537, 46.5432) ccw projected
  circle A42 centre (60.6166, -3.0869) radius 1.5 projected
  line L24 (60.6166, -3.0869) -> (51.7652, -11.1896)
  line L25 (56.1909, -7.1382) -> (46.0625, 3.9259)
  line L26 (38.7245, -2.868) -> (52.1909, -17.5786) projected
  line L27 (43.3616, 6.8764) -> (48.7634, 0.9755) construction
  line L28 (39.6736, 3.5003) -> (45.0754, -2.4006)
  line L29 (52.4515, 4.3516) -> (47.0497, 10.2525)
  arc A43 (47.0497, 10.2525) -> (39.6736, 3.5003) centre (43.3616, 6.8764) ccw
  arc A44 (45.0754, -2.4006) -> (52.4515, 4.3516) centre (48.7634, 0.9755) ccw
  dimension "d77" = 15
  dimension "d78" = 4
  dimension "d79" = 10
  constraints: 12 end point, 4 point on circle, 4 tangent, 2 centre point, 2 midpoint, 2 parallel, 1 point on line
  measures "d77" distance of L25.start L25.end
  measures "d78" distance of L25.end L27.end
  measures "d79" diameter of A44
extrude "Extrusion11" cut sketch "Sketch13" against normal blind 10 contours A43 L29 A44 L28
sketch "Sketch14" plane through (0, 0, 8) normal (0, 0, 1) x (1, 0, 0)
  line L0 (47.0497, 10.2525) -> (52.4515, 4.3516) projected
  arc A0 (45.0754, -2.4006) -> (52.4515, 4.3516) centre (48.7634, 0.9755) ccw projected
  line L1 (45.0754, -2.4006) -> (39.6736, 3.5003) projected
  arc A1 (47.0497, 10.2525) -> (39.6736, 3.5003) centre (43.3616, 6.8764) ccw projected
  circle A2 centre (-7.332, -16.439) radius 1.5 projected
  circle A3 centre (17.9975, 0.3024) radius 1.5 projected
  circle A4 centre (-0.3024, 17.9975) radius 1.5 projected
  circle A5 centre (105.9874, 42.242) radius 1.5 projected
  circle A6 centre (81.2775, 54.469) radius 1.5 projected
  circle A7 centre (82.6991, 28.6391) radius 1.5 projected
  circle A8 centre (0, 0) radius 6.5 projected
  circle A9 centre (28.3096, 63.473) radius 8 projected
  circle A10 centre (94.4874, 42.242) radius 8 projected
  circle A11 centre (54.9885, 62.7904) radius 2 projected
  circle A12 centre (68.3193, 58.5137) radius 2 projected
  arc A13 (38.5327, 52.4963) -> (41.9543, 57.2422) centre (28.3096, 63.473) ccw projected
  arc A14 (44.3846, 58.3158) -> (41.9543, 57.2422) centre (43.7736, 56.4114) ccw projected
  line L2 (44.3846, 58.3158) -> (78.4124, 47.3991) projected
  arc A15 (79.7645, 45.112) -> (78.4124, 47.3991) centre (77.8015, 45.4947) ccw projected
  arc A16 (79.7645, 45.112) -> (80.1684, 37.7735) centre (94.4874, 42.242) ccw projected
  arc A17 (79.0755, 35.3519) -> (80.1684, 37.7735) centre (78.2592, 37.1777) ccw projected
  line L3 (79.0755, 35.3519) -> (54.0906, 24.182) projected
  arc A18 (48.8064, 26.2012) -> (54.0906, 24.182) centre (52.4581, 27.8337) ccw projected
  line L4 (48.8064, 26.2012) -> (38.07, 50.2164) projected
  arc A19 (38.5327, 52.4963) -> (38.07, 50.2164) centre (39.8958, 51.0327) ccw projected
  circle A20 centre (-23.6864, 10.4368) radius 1.5 projected
  circle A21 centre (23.5915, -10.6496) radius 1.5 projected
  circle A22 centre (-10.5906, -23.7453) radius 1.5 projected
  circle A23 centre (60.6166, -3.0869) radius 1.5 projected
  circle A24 centre (51.7652, -11.1896) radius 1.5 projected
  line L5 (27.2264, -6.796) -> (28.2383, -9.4372) projected
  arc A25 (29.5934, -3.2006) -> (27.2264, -6.796) centre (31.226, -6.8523) ccw projected
  line L6 (29.5934, -3.2006) -> (32.9958, -1.6795) projected
  arc A26 (38.7245, -2.868) -> (32.9958, -1.6795) centre (35.0365, -6.2441) ccw projected
  line L7 (38.7245, -2.868) -> (52.1909, -17.5786) projected
  line L8 (52.1909, -17.5786) -> (66.9432, -4.074) projected
  line L9 (66.9432, -4.074) -> (58.3371, 5.3271) projected
  arc A27 (59.3255, 10.0916) -> (58.3371, 5.3271) centre (60.5499, 7.3528) ccw projected
  line L10 (59.3255, 10.0916) -> (100.6094, 28.5482) projected
  arc A28 (100.6094, 28.5482) -> (99.0696, 56.525) centre (94.4874, 42.242) ccw projected
  line L11 (99.0696, 56.525) -> (32.8918, 77.7559) projected
  arc A29 (32.8918, 77.7559) -> (14.6104, 69.5829) centre (28.3096, 63.473) ccw projected
  line L12 (14.6104, 69.5829) -> (-10.0806, 14.2231) projected
  arc A30 (-15.3631, 12.1994) -> (-10.0806, 14.2231) centre (-13.7338, 15.8525) ccw projected
  line L13 (-15.3631, 12.1994) -> (-23.2479, 15.7161) projected
  line L14 (-25.8892, 14.7042) -> (-23.2479, 15.7161) projected
  line L15 (-25.8892, 14.7042) -> (-29.1478, 7.3979) projected
  line L16 (-29.1478, 7.3979) -> (-17.3085, 2.1175) projected
  arc A31 (-14.9509, -1.2123) -> (-17.3085, 2.1175) centre (-18.9378, -1.5356) ccw projected
  arc A32 (-14.9509, -1.2123) -> (-11.8701, -9.1706) centre (0, 0) ccw projected
  arc A33 (-11.3824, -13.2454) -> (-11.8701, -9.1706) centre (-15.0355, -11.6161) ccw projected
  line L17 (-11.3824, -13.2454) -> (-16.6845, -25.1334) projected
  line L18 (-16.6845, -25.1334) -> (-7.5517, -29.2067) projected
  line L19 (-7.5517, -29.2067) -> (-2.2496, -17.3188) projected
  arc A34 (1.1081, -14.959) -> (-2.2496, -17.3188) centre (1.4035, -18.9481) ccw projected
  arc A35 (1.1081, -14.959) -> (6.122, -13.6938) centre (0, 0) ccw projected
  line L20 (6.122, -13.6938) -> (10.4943, -11.7391) projected
  arc A36 (13.7562, -11.7377) -> (10.4943, -11.7391) centre (12.1268, -15.3908) ccw projected
  line L21 (13.7562, -11.7377) -> (24.9796, -16.7435) projected
  line L22 (24.9796, -16.7435) -> (28.2383, -9.4372) projected
  line L23 (31.6795, 47.3595) -> (42.4159, 23.3442) projected
  arc A37 (40.3968, 18.06) -> (42.4159, 23.3442) centre (38.7642, 21.7117) ccw projected
  line L24 (40.3968, 18.06) -> (15.4119, 6.8901) projected
  arc A38 (12.8785, 7.6905) -> (15.4119, 6.8901) centre (14.5956, 8.716) ccw projected
  arc A39 (12.8785, 7.6905) -> (7.6792, 12.8852) centre (0, 0) ccw projected
  arc A40 (6.8766, 15.4179) -> (7.6792, 12.8852) centre (8.7031, 14.6033) ccw projected
  line L25 (6.8766, 15.4179) -> (21.4331, 48.055) projected
  arc A41 (23.8537, 49.1501) -> (21.4331, 48.055) centre (23.2596, 47.2403) ccw projected
  arc A42 (23.8537, 49.1501) -> (29.672, 48.535) centre (28.3096, 63.473) ccw projected
  arc A43 (31.6795, 47.3595) -> (29.672, 48.535) centre (29.8537, 46.5432) ccw projected
  circle A44 centre (82.6991, 28.6391) radius 1.5 projected
  circle A45 centre (17.9975, 0.3024) radius 1.5 projected
  line L26 (82.6991, 28.6391) -> (17.9975, 0.3024)
  line L27 (17.9975, 0.3024) -> (25.3255, 3.5118)
  line L28 (25.3255, 3.5118) -> (30.8215, 5.9188) construction
  line L29 (26.3284, 1.2218) -> (31.8244, 3.6288)
  line L30 (29.8186, 8.2088) -> (24.3225, 5.8018)
  arc A46 (24.3225, 5.8018) -> (26.3284, 1.2218) centre (25.3255, 3.5118) ccw
  arc A47 (31.8244, 3.6288) -> (29.8186, 8.2088) centre (30.8215, 5.9188) ccw
  line L31 (82.6991, 28.6391) -> (74.4551, 25.0286)
  line L32 (74.4551, 25.0286) -> (68.0431, 22.2204) construction
  line L33 (73.4522, 27.3186) -> (67.0402, 24.5104)
  line L34 (69.046, 19.9304) -> (75.458, 22.7386)
  arc A48 (75.458, 22.7386) -> (73.4522, 27.3186) centre (74.4551, 25.0286) ccw
  arc A49 (67.0402, 24.5104) -> (69.046, 19.9304) centre (68.0431, 22.2204) ccw
  line L35 (68.0431, 22.2204) -> (58.8831, 18.2087)
  line L36 (58.8831, 18.2087) -> (52.471, 15.4005) construction
  line L37 (57.8801, 20.4987) -> (51.4681, 17.6905)
  line L38 (53.474, 13.1104) -> (59.886, 15.9187)
  arc A50 (59.886, 15.9187) -> (57.8801, 20.4987) centre (58.8831, 18.2087) ccw
  arc A51 (51.4681, 17.6905) -> (53.474, 13.1104) centre (52.471, 15.4005) ccw
  point P0 (28.0735, 4.7153)
  point P1 (71.2491, 23.6245)
  point P2 (55.6771, 16.8046)
  dimension "d82" = 8
  dimension "d83" = 6
  dimension "d84" = 5
  dimension "d85" = 9
  dimension "d86" = 7
  dimension "d87" = 5
  dimension "d88" = 10
  dimension "d89" = 7
  dimension "d90" = 5
  constraints: 32 end point, 12 point on circle, 12 tangent, 6 centre point, 6 point on line, 3 midpoint, 3 parallel
  measures "d82" distance of L26.end L27.end
  measures "d83" distance of L27.end L28.end
  measures "d84" diameter of A47
  measures "d85" distance of L26.start L31.end
  measures "d86" distance of L31.end L32.end
  measures "d87" diameter of A49
  measures "d88" distance of L32.end L35.end
  measures "d89" distance of L35.end L36.end
  measures "d90" diameter of A51
extrude "Extrusion12" cut sketch "Sketch14" against normal blind 10 contours L26 A48 L34 A49 | L26 A49 L33 A48 | A50 L38 A51 L26 | L26 A51 L37 A50 | A47 L29 A46 L26 | L26 A46 L30 A47
sketch "Sketch15" plane through (0, 0, 8) normal (0, 0, 1) x (1, 0, 0)
  arc A0 (31.8244, 3.6288) -> (29.8186, 8.2088) centre (30.8215, 5.9188) ccw projected
  line L0 (31.8244, 3.6288) -> (26.3284, 1.2218) projected
  arc A1 (24.3225, 5.8018) -> (26.3284, 1.2218) centre (25.3255, 3.5118) ccw projected
  line L1 (24.3225, 5.8018) -> (29.8186, 8.2088) projected
  arc A2 (51.4681, 17.6905) -> (53.474, 13.1104) centre (52.471, 15.4005) ccw projected
  line L2 (51.4681, 17.6905) -> (57.8801, 20.4987) projected
  arc A3 (59.886, 15.9187) -> (57.8801, 20.4987) centre (58.8831, 18.2087) ccw projected
  line L3 (59.886, 15.9187) -> (53.474, 13.1104) projected
  line L4 (67.0402, 24.5104) -> (73.4522, 27.3186) projected
  arc A4 (75.458, 22.7386) -> (73.4522, 27.3186) centre (74.4551, 25.0286) ccw projected
  line L5 (75.458, 22.7386) -> (69.046, 19.9304) projected
  arc A5 (67.0402, 24.5104) -> (69.046, 19.9304) centre (68.0431, 22.2204) ccw projected
  line L6 (47.0497, 10.2525) -> (52.4515, 4.3516) projected
  arc A6 (45.0754, -2.4006) -> (52.4515, 4.3516) centre (48.7634, 0.9755) ccw projected
  line L7 (45.0754, -2.4006) -> (39.6736, 3.5003) projected
  arc A7 (47.0497, 10.2525) -> (39.6736, 3.5003) centre (43.3616, 6.8764) ccw projected
  circle A8 centre (-7.332, -16.439) radius 1.5 projected
  circle A9 centre (17.9975, 0.3024) radius 1.5 projected
  circle A10 centre (-0.3024, 17.9975) radius 1.5 projected
  circle A11 centre (105.9874, 42.242) radius 1.5 projected
  circle A12 centre (81.2775, 54.469) radius 1.5 projected
  circle A13 centre (82.6991, 28.6391) radius 1.5 projected
  circle A14 centre (0, 0) radius 6.5 projected
  circle A15 centre (28.3096, 63.473) radius 8 projected
  circle A16 centre (94.4874, 42.242) radius 8 projected
  circle A17 centre (54.9885, 62.7904) radius 2 projected
  circle A18 centre (68.3193, 58.5137) radius 2 projected
  arc A19 (38.5327, 52.4963) -> (41.9543, 57.2422) centre (28.3096, 63.473) ccw projected
  arc A20 (44.3846, 58.3158) -> (41.9543, 57.2422) centre (43.7736, 56.4114) ccw projected
  line L8 (44.3846, 58.3158) -> (78.4124, 47.3991) projected
  arc A21 (79.7645, 45.112) -> (78.4124, 47.3991) centre (77.8015, 45.4947) ccw projected
  arc A22 (79.7645, 45.112) -> (80.1684, 37.7735) centre (94.4874, 42.242) ccw projected
  arc A23 (79.0755, 35.3519) -> (80.1684, 37.7735) centre (78.2592, 37.1777) ccw projected
  line L9 (79.0755, 35.3519) -> (54.0906, 24.182) projected
  arc A24 (48.8064, 26.2012) -> (54.0906, 24.182) centre (52.4581, 27.8337) ccw projected
  line L10 (48.8064, 26.2012) -> (38.07, 50.2164) projected
  arc A25 (38.5327, 52.4963) -> (38.07, 50.2164) centre (39.8958, 51.0327) ccw projected
  circle A26 centre (-23.6864, 10.4368) radius 1.5 projected
  circle A27 centre (23.5915, -10.6496) radius 1.5 projected
  circle A28 centre (-10.5906, -23.7453) radius 1.5 projected
  circle A29 centre (60.6166, -3.0869) radius 1.5 projected
  circle A30 centre (51.7652, -11.1896) radius 1.5 projected
  line L11 (27.2264, -6.796) -> (28.2383, -9.4372) projected
  arc A31 (29.5934, -3.2006) -> (27.2264, -6.796) centre (31.226, -6.8523) ccw projected
  line L12 (29.5934, -3.2006) -> (32.9958, -1.6795) projected
  arc A32 (38.7245, -2.868) -> (32.9958, -1.6795) centre (35.0365, -6.2441) ccw projected
  line L13 (38.7245, -2.868) -> (52.1909, -17.5786) projected
  line L14 (52.1909, -17.5786) -> (66.9432, -4.074) projected
  line L15 (66.9432, -4.074) -> (58.3371, 5.3271) projected
  arc A33 (59.3255, 10.0916) -> (58.3371, 5.3271) centre (60.5499, 7.3528) ccw projected
  line L16 (59.3255, 10.0916) -> (100.6094, 28.5482) projected
  arc A34 (100.6094, 28.5482) -> (99.0696, 56.525) centre (94.4874, 42.242) ccw projected
  line L17 (99.0696, 56.525) -> (32.8918, 77.7559) projected
  arc A35 (32.8918, 77.7559) -> (14.6104, 69.5829) centre (28.3096, 63.473) ccw projected
  line L18 (14.6104, 69.5829) -> (-10.0806, 14.2231) projected
  arc A36 (-15.3631, 12.1994) -> (-10.0806, 14.2231) centre (-13.7338, 15.8525) ccw projected
  line L19 (-15.3631, 12.1994) -> (-23.2479, 15.7161) projected
  line L20 (-25.8892, 14.7042) -> (-23.2479, 15.7161) projected
  line L21 (-25.8892, 14.7042) -> (-29.1478, 7.3979) projected
  line L22 (-29.1478, 7.3979) -> (-17.3085, 2.1175) projected
  arc A37 (-14.9509, -1.2123) -> (-17.3085, 2.1175) centre (-18.9378, -1.5356) ccw projected
  arc A38 (-14.9509, -1.2123) -> (-11.8701, -9.1706) centre (0, 0) ccw projected
  arc A39 (-11.3824, -13.2454) -> (-11.8701, -9.1706) centre (-15.0355, -11.6161) ccw projected
  line L23 (-11.3824, -13.2454) -> (-16.6845, -25.1334) projected
  line L24 (-16.6845, -25.1334) -> (-7.5517, -29.2067) projected
  line L25 (-7.5517, -29.2067) -> (-2.2496, -17.3188) projected
  arc A40 (1.1081, -14.959) -> (-2.2496, -17.3188) centre (1.4035, -18.9481) ccw projected
  arc A41 (1.1081, -14.959) -> (6.122, -13.6938) centre (0, 0) ccw projected
  line L26 (6.122, -13.6938) -> (10.4943, -11.7391) projected
  arc A42 (13.7562, -11.7377) -> (10.4943, -11.7391) centre (12.1268, -15.3908) ccw projected
  line L27 (13.7562, -11.7377) -> (24.9796, -16.7435) projected
  line L28 (24.9796, -16.7435) -> (28.2383, -9.4372) projected
  line L29 (31.6795, 47.3595) -> (42.4159, 23.3442) projected
  arc A43 (40.3968, 18.06) -> (42.4159, 23.3442) centre (38.7642, 21.7117) ccw projected
  line L30 (40.3968, 18.06) -> (15.4119, 6.8901) projected
  arc A44 (12.8785, 7.6905) -> (15.4119, 6.8901) centre (14.5956, 8.716) ccw projected
  arc A45 (12.8785, 7.6905) -> (7.6792, 12.8852) centre (0, 0) ccw projected
  arc A46 (6.8766, 15.4179) -> (7.6792, 12.8852) centre (8.7031, 14.6033) ccw projected
  line L31 (6.8766, 15.4179) -> (21.4331, 48.055) projected
  arc A47 (23.8537, 49.1501) -> (21.4331, 48.055) centre (23.2596, 47.2403) ccw projected
  arc A48 (23.8537, 49.1501) -> (29.672, 48.535) centre (28.3096, 63.473) ccw projected
  arc A49 (31.6795, 47.3595) -> (29.672, 48.535) centre (29.8537, 46.5432) ccw projected
  circle A50 centre (-0.3024, 17.9975) radius 1.5 projected
  line L32 (-0.3024, 17.9975) -> (3.7709, 27.1303)
  line L33 (14.6104, 69.5829) -> (-10.0806, 14.2231) projected
  line L34 (3.7709, 27.1303) -> (7.0296, 34.4365) construction
  line L35 (6.0541, 26.1119) -> (9.3128, 33.4182)
  line L36 (4.7464, 35.4548) -> (1.4877, 28.1486)
  arc A51 (1.4877, 28.1486) -> (6.0541, 26.1119) centre (3.7709, 27.1303) ccw
  arc A52 (9.3128, 33.4182) -> (4.7464, 35.4548) centre (7.0296, 34.4365) ccw
  line L37 (7.0296, 34.4365) -> (11.9176, 45.3959)
  line L38 (11.9176, 45.3959) -> (15.1762, 52.7021) construction
  line L39 (14.2008, 44.3775) -> (17.4594, 51.6838)
  line L40 (12.893, 53.7204) -> (9.6344, 46.4142)
  arc A53 (9.6344, 46.4142) -> (14.2008, 44.3775) centre (11.9176, 45.3959) ccw
  arc A54 (17.4594, 51.6838) -> (12.893, 53.7204) centre (15.1762, 52.7021) ccw
  point P0 (5.4003, 30.7834)
  point P1 (13.5469, 49.049)
  dimension "d93" = 10
  dimension "d94" = 8
  dimension "d95" = 5
  dimension "d96" = 12
  dimension "d97" = 8
  dimension "d98" = 5
  constraints: 20 end point, 8 point on circle, 8 tangent, 6 parallel, 4 centre point, 2 midpoint
  measures "d93" distance of L32.start L32.end
  measures "d94" distance of L32.end L34.end
  measures "d95" diameter of A52
  measures "d96" distance of L34.end L37.end
  measures "d97" distance of L37.end L38.end
  measures "d98" diameter of A54
extrude "Extrusion13" cut sketch "Sketch15" against normal blind 10 contours A51 L36 A52 L35 | A53 L40 A54 L39
body "Solid1"
